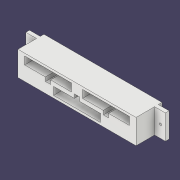
# Autodesk Inventor part: BP011
Saved by Autodesk Inventor 2017 SP1 (Build 210196100, 196)
## iProperties
Created: 2018-06-18
Part Number: BP011
Material: ABS Plastic
Document SubType Name: Modeling
Designer: Zach
Density: 1.06 g/cm^3
Appearance: CR White
Author: Zach
Autodesk Inventor part; units mm, degrees
ref_plane "YZ Plane" through (0, 0, 0) normal (1, 0, 0) x (0, 1, 0)
ref_plane "XZ Plane" through (0, 0, 0) normal (0, 1, 0) x (-1, 0, 0)
ref_plane "XY Plane" through (0, 0, 0) normal (0, 0, 1) x (1, 0, 0)
sketch "Sketch1" plane through (0, 0, 0) normal (0, 0, 1) x (1, 0, 0)
  line L0 (0, 0) -> (190, 0)
  line L1 (190, 0) -> (190, 35)
  line L2 (190, 35) -> (0, 35)
  line L3 (0, 35) -> (0, 0)
  circle A0 centre (7.5, 17.5) radius 1.5
  circle A1 centre (182.5, 17.5) radius 1.5
  point P0 (0, 17.5)
  dimension "d0" = 190
  dimension "d1" = 35
  dimension "d2" = 3
  dimension "d3" = 7.5
  dimension "d4" = 3
  dimension "d5" = 7.5
  constraints: 8 end point, 2 centre point, 2 horizontal alignment, 2 parallel, 1 horizontal, 1 midpoint, 1 perpendicular
  measures "d0" distance of L2.end L1.end
  measures "d1" distance of L1.end L0.end
  measures "d2" diameter of A0
  measures "d3" distance from line of L3 A0.centre
  measures "d4" diameter of A1
  measures "d5" distance from line of L1 A1.centre
extrude "Extrusion1" add sketch "Sketch1" along normal blind 5
sketch "Sketch2" plane through (0, 0, 0) normal (0, 0, -1) x (-1, 0, 0)
  line L0 (0, 0) -> (-190, 0) projected
  line L1 (-190, 35) -> (0, 35) projected
  line L2 (-15.5, 0) -> (-174.5, 0)
  line L3 (-174.5, 0) -> (-174.5, 35)
  line L4 (-174.5, 35) -> (-15.5, 35)
  line L5 (-15.5, 35) -> (-15.5, 0)
  point P0 (-95, 0)
  dimension "d8" = 159
  constraints: 8 end point, 2 midpoint, 2 parallel, 2 point on line, 1 horizontal, 1 perpendicular
  measures "d8" distance between parallel lines of L5 L3
extrude "Extrusion2" add sketch "Sketch2" along normal blind 5
sketch "Sketch3" plane through (0, 0, 5) normal (0, 0, 1) x (1, 0, 0)
  circle A0 centre (182.5, 17.5) radius 1.5 projected
  circle A1 centre (7.5, 17.5) radius 1.5 projected
  line L0 (0, 0) -> (190, 0) projected
  line L1 (190, 0) -> (190, 35) projected
  line L2 (190, 35) -> (0, 35) projected
  line L3 (0, 35) -> (0, 0) projected
  line L4 (1, 34) -> (189, 34)
  line L5 (189, 34) -> (189, 1)
  line L6 (189, 1) -> (1, 1)
  line L7 (1, 1) -> (1, 34)
  dimension "d11" = 1
  constraints: 8 end point, 3 other
  measures "d11" distance between parallel lines of L2 L4
extrude "Extrusion3" cut sketch "Sketch3" against normal through all contours L3 L2 L1 L0
sketch "Sketch4" plane through (0, 0, 5) normal (0, 0, 1) x (1, 0, 0)
  line L0 (41, 27) -> (71, 27)
  line L1 (71, 27) -> (71, 8)
  line L2 (71, 8) -> (41, 8)
  line L3 (41, 8) -> (41, 27)
  line L4 (86, 27) -> (116, 27)
  line L5 (116, 27) -> (116, 8)
  line L6 (116, 8) -> (86, 8)
  line L7 (86, 8) -> (86, 27)
  line L8 (131, 27) -> (149, 27)
  line L9 (149, 27) -> (149, 8)
  line L10 (149, 8) -> (131, 8)
  line L11 (131, 8) -> (131, 27)
  line L12 (41, 17.5) -> (149, 17.5) construction
  line L13 (189, 34) -> (1, 34) projected
  circle A0 centre (7.5, 17.5) radius 1.5 projected
  point P0 (0, 0)
  point P1 (95, 17.5)
  point P2 (95, 34)
  dimension "d14" = 30
  dimension "d15" = 19
  dimension "d16" = 30
  dimension "d17" = 19
  dimension "d18" = 18
  dimension "d19" = 19
  dimension "d20" = 15
  dimension "d21" = 15
  constraints: 26 end point, 6 parallel, 4 midpoint, 3 horizontal, 3 perpendicular, 2 point on line, 1 horizontal alignment, 1 vertical alignment
  measures "d14" distance of L1.end L2.end
  measures "d15" distance of L0.end L1.end
  measures "d16" distance of L5.end L6.end
  measures "d17" distance of L4.end L5.end
  measures "d18" distance of L9.end L10.end
  measures "d19" distance of L8.end L9.end
  measures "d20" distance between parallel lines of L1 L7
  measures "d21" distance between parallel lines of L11 L5
extrude "Extrusion4" cut sketch "Sketch4" against normal through all contours L0 L1 L2 L3 | L4 L5 L6 L7 | L8 L9 L10 L11
sketch "Sketch5" plane through (0, 0, 5) normal (0, 0, 1) x (1, 0, 0)
  line L0 (41, 27) -> (41, 8) projected
  line L1 (41, 8) -> (71, 8) projected
  line L2 (71, 8) -> (71, 27) projected
  line L3 (71, 27) -> (41, 27) projected
  line L4 (131, 27) -> (131, 8) projected
  line L5 (131, 8) -> (149, 8) projected
  line L6 (149, 8) -> (149, 27) projected
  line L7 (149, 27) -> (131, 27) projected
  line L8 (86, 27) -> (86, 8) projected
  line L9 (86, 8) -> (116, 8) projected
  line L10 (116, 8) -> (116, 27) projected
  line L11 (116, 27) -> (86, 27) projected
  line L12 (174.5, 1) -> (15.5, 1) projected
  line L13 (15.5, 1) -> (15.5, 34) projected
  line L14 (15.5, 34) -> (174.5, 34) projected
  line L15 (174.5, 34) -> (174.5, 1) projected
  point P0 (0, 0)
extrude "Extrusion5" add sketch "Sketch5" along normal blind 25
sketch "Sketch6" plane through (0, 0, -5) normal (0, 0, -1) x (-1, 0, 0)
  line L0 (-71, 27) -> (-41, 27) projected
  line L1 (-41, 27) -> (-41, 8) projected
  line L2 (-71, 8) -> (-71, 27) projected
  line L3 (-86, 27) -> (-86, 8) projected
  line L4 (-116, 27) -> (-86, 27) projected
  line L5 (-116, 8) -> (-116, 27) projected
  line L6 (-41, 25) -> (-36, 25)
  line L7 (-36, 25) -> (-36, 10)
  line L8 (-36, 10) -> (-41, 10)
  line L9 (-41, 10) -> (-41, 25)
  line L10 (-71, 25) -> (-76, 25)
  line L11 (-76, 25) -> (-76, 10)
  line L12 (-76, 10) -> (-71, 10)
  line L13 (-71, 10) -> (-71, 25)
  line L14 (-86, 25) -> (-81, 25)
  line L15 (-81, 25) -> (-81, 10)
  line L16 (-81, 10) -> (-86, 10)
  line L17 (-86, 10) -> (-86, 25)
  line L18 (-116, 25) -> (-121, 25)
  line L19 (-121, 25) -> (-121, 10)
  line L20 (-121, 10) -> (-116, 10)
  line L21 (-116, 10) -> (-116, 25)
  point P0 (0, 0)
  point P1 (-41, 17.5)
  dimension "d26" = 15
  dimension "d27" = 5
  dimension "d28" = 5
  dimension "d29" = 5
  dimension "d30" = 5
  constraints: 32 end point, 8 parallel, 6 horizontal alignment, 4 horizontal, 4 perpendicular, 4 point on line, 2 midpoint
  measures "d26" distance of L6.end L7.end
  measures "d27" distance of L6.start L6.end
  measures "d28" distance of L10.start L10.end
  measures "d29" distance of L14.start L14.end
  measures "d30" distance of L18.start L18.end
extrude "Extrusion6" cut sketch "Sketch6" against normal blind 22
sketch "Sketch10" plane through (0, 0, 30) normal (0, 0, 1) x (1, 0, 0)
  line L0 (86, 27) -> (116, 27) projected
  line L1 (116, 27) -> (116, 8) projected
  line L2 (116, 8) -> (86, 8) projected
  line L3 (86, 8) -> (86, 27) projected
  line L4 (41, 27) -> (71, 27) projected
  line L5 (71, 27) -> (71, 8) projected
  line L6 (71, 8) -> (41, 8) projected
  line L7 (41, 8) -> (41, 27) projected
  line L8 (131, 27) -> (149, 27) projected
  line L9 (149, 27) -> (149, 8) projected
  line L10 (149, 8) -> (131, 8) projected
  line L11 (131, 8) -> (131, 27) projected
  line L12 (15.5, 1) -> (174.5, 1) projected
  line L13 (174.5, 1) -> (174.5, 34) projected
  line L14 (174.5, 34) -> (15.5, 34) projected
  line L15 (15.5, 34) -> (15.5, 1) projected
  point P0 (0, 0)
extrude "Extrusion7" add sketch "Sketch10" against normal blind 35 contours L0 L1 L2 L3 | L4 L5 L6 L7 | L8 L9 L10 L11 | L15 L14 L13 L12
sketch "Sketch11" plane through (0, 0, 30) normal (0, 0, 1) x (1, 0, 0)
  line L0 (29.5, 32) -> (82.5, 32)
  line L1 (82.5, 32) -> (82.5, 19)
  line L2 (82.5, 19) -> (29.5, 19)
  line L3 (29.5, 19) -> (29.5, 32)
  line L4 (107.5, 32) -> (160.5, 32)
  line L5 (160.5, 32) -> (160.5, 19)
  line L6 (160.5, 19) -> (107.5, 19)
  line L7 (107.5, 19) -> (107.5, 32)
  line L8 (29.5, 32) -> (160.5, 32)
  line L9 (174.5, 34) -> (15.5, 34) projected
  line L10 (29.5, 32) -> (29.5, 3)
  line L11 (15.5, 34) -> (15.5, 1) projected
  line L12 (52.5, 19) -> (59.5, 19)
  line L13 (59.5, 19) -> (59.5, 15)
  line L14 (59.5, 15) -> (52.5, 15)
  line L15 (52.5, 15) -> (52.5, 19)
  line L16 (130.5, 19) -> (137.5, 19)
  line L17 (137.5, 19) -> (137.5, 15)
  line L18 (137.5, 15) -> (130.5, 15)
  line L19 (130.5, 15) -> (130.5, 19)
  line L20 (68.5, 3) -> (121.5, 3)
  line L21 (121.5, 3) -> (121.5, 16)
  line L22 (121.5, 16) -> (68.5, 16)
  line L23 (68.5, 16) -> (68.5, 3)
  line L24 (91.5, 16) -> (98.5, 16)
  line L25 (98.5, 16) -> (98.5, 20)
  line L26 (98.5, 20) -> (91.5, 20)
  line L27 (91.5, 20) -> (91.5, 16)
  point P0 (0, 0)
  point P1 (95, 32)
  point P2 (95, 34)
  point P3 (29.5, 17.5)
  point P4 (15.5, 17.5)
  point P5 (56, 19)
  point P6 (134, 19)
  point P7 (95, 16)
  point P8 (95, 20)
  dimension "d40" = 53
  dimension "d41" = 13
  dimension "d42" = 53
  dimension "d43" = 13
  dimension "d46" = 25
  dimension "d48" = 7
  dimension "d49" = 7
  dimension "d50" = 4
  dimension "d53" = 53
  dimension "d54" = 13
  dimension "d55" = 7
  dimension "d56" = 4
  dimension "d57" = 3
  dimension "d58" = 4
  constraints: 52 end point, 12 parallel, 11 midpoint, 6 horizontal, 6 perpendicular, 4 point on line, 3 horizontal alignment, 2 vertical alignment
  measures "d40" distance of L1.end L2.end
  measures "d41" distance of L2.end L0.start
  measures "d42" distance of L5.end L6.end
  measures "d43" distance of L6.end L4.start
  measures "d46" distance between parallel lines of L7 L1
  measures "d48" distance between parallel lines of L15 L13
  measures "d49" distance of L17.end L18.end
  measures "d50" distance of L16.end L17.end
  measures "d53" distance of L22.end L21.end
  measures "d54" distance of L21.end L20.end
  measures "d55" distance of L26.end L25.end
  measures "d56" distance of L25.end L24.end
  measures "d57" distance between parallel lines of L2 L22
  measures "d58" distance of L14.end L12.start
extrude "Extrusion8" cut sketch "Sketch11" against normal through all
sketch "Sketch13" plane through (0, 0, 30) normal (0, 0, 1) x (1, 0, 0)
  line L0 (98.5, 16) -> (121.5, 16) projected
  line L1 (121.5, 16) -> (121.5, 3) projected
  line L2 (121.5, 3) -> (68.5, 3) projected
  line L3 (68.5, 3) -> (68.5, 16) projected
  line L4 (68.5, 16) -> (91.5, 16) projected
  line L5 (91.5, 16) -> (91.5, 20) projected
  line L6 (91.5, 20) -> (98.5, 20) projected
  line L7 (98.5, 20) -> (98.5, 16) projected
  line L8 (52.5, 19) -> (29.5, 19) projected
  line L9 (29.5, 19) -> (29.5, 32) projected
  line L10 (29.5, 32) -> (82.5, 32) projected
  line L11 (82.5, 32) -> (82.5, 19) projected
  line L12 (82.5, 19) -> (59.5, 19) projected
  line L13 (59.5, 19) -> (59.5, 15) projected
  line L14 (59.5, 15) -> (52.5, 15) projected
  line L15 (52.5, 15) -> (52.5, 19) projected
  line L16 (130.5, 19) -> (107.5, 19) projected
  line L17 (107.5, 19) -> (107.5, 32) projected
  line L18 (107.5, 32) -> (160.5, 32) projected
  line L19 (160.5, 32) -> (160.5, 19) projected
  line L20 (160.5, 19) -> (137.5, 19) projected
  line L21 (137.5, 19) -> (137.5, 15) projected
  line L22 (137.5, 15) -> (130.5, 15) projected
  line L23 (130.5, 15) -> (130.5, 19) projected
  line L24 (15.5, 1) -> (174.5, 1) projected
  line L25 (174.5, 1) -> (174.5, 34) projected
  line L26 (174.5, 34) -> (15.5, 34) projected
  line L27 (15.5, 34) -> (15.5, 1) projected
  point P0 (0, 0)
extrude "Extrusion10" cut sketch "Sketch13" against normal blind 25
sketch "Sketch12" plane through (0, 0, 5) normal (0, 0, 1) x (1, 0, 0)
  line L0 (29.5, 19) -> (29.5, 32)
  line L1 (82.5, 32) -> (82.5, 19)
  line L2 (29.5, 30.75) -> (82.5, 30.75)
  line L3 (82.5, 30.75) -> (82.5, 20.25)
  line L4 (82.5, 20.25) -> (29.5, 20.25)
  line L5 (29.5, 20.25) -> (29.5, 30.75)
  line L6 (107.5, 19) -> (107.5, 32)
  line L7 (160.5, 19) -> (160.5, 32)
  line L8 (107.5, 30.75) -> (160.5, 30.75)
  line L9 (160.5, 30.75) -> (160.5, 20.25)
  line L10 (160.5, 20.25) -> (107.5, 20.25)
  line L11 (107.5, 20.25) -> (107.5, 30.75)
  line L12 (121.5, 3) -> (121.5, 16)
  line L13 (121.5, 14.75) -> (68.5, 14.75)
  line L14 (68.5, 14.75) -> (68.5, 4.25)
  line L15 (68.5, 4.25) -> (121.5, 4.25)
  line L16 (121.5, 4.25) -> (121.5, 14.75)
  line L17 (68.5, 3) -> (68.5, 16)
  line L18 (98.5, 16) -> (121.5, 16)
  line L19 (121.5, 16) -> (121.5, 3)
  line L20 (121.5, 3) -> (68.5, 3)
  line L21 (68.5, 3) -> (68.5, 16)
  line L22 (68.5, 16) -> (91.5, 16)
  line L23 (91.5, 16) -> (91.5, 20)
  line L24 (91.5, 20) -> (98.5, 20)
  line L25 (98.5, 20) -> (98.5, 16)
  line L26 (52.5, 19) -> (29.5, 19)
  line L27 (29.5, 19) -> (29.5, 32)
  line L28 (29.5, 32) -> (82.5, 32)
  line L29 (82.5, 32) -> (82.5, 19)
  line L30 (82.5, 19) -> (59.5, 19)
  line L31 (59.5, 19) -> (59.5, 15)
  line L32 (59.5, 15) -> (52.5, 15)
  line L33 (52.5, 15) -> (52.5, 19)
  line L34 (130.5, 19) -> (107.5, 19)
  line L35 (107.5, 19) -> (107.5, 32)
  line L36 (107.5, 32) -> (160.5, 32)
  line L37 (160.5, 32) -> (160.5, 19)
  line L38 (160.5, 19) -> (137.5, 19)
  line L39 (137.5, 19) -> (137.5, 15)
  line L40 (137.5, 15) -> (130.5, 15)
  line L41 (130.5, 15) -> (130.5, 19)
  line L42 (15.5, 1) -> (174.5, 1)
  line L43 (174.5, 1) -> (174.5, 34)
  line L44 (174.5, 34) -> (15.5, 34)
  line L45 (15.5, 34) -> (15.5, 1)
  line L46 (98.5, 16) -> (98.5, 20)
  line L47 (91.5, 14.75) -> (98.5, 14.75)
  line L48 (98.5, 14.75) -> (98.5, 20)
  line L49 (98.5, 20) -> (91.5, 20)
  line L50 (91.5, 20) -> (91.5, 14.75)
  line L51 (52.5, 19) -> (52.5, 15)
  line L52 (52.5, 15) -> (59.5, 15)
  line L53 (59.5, 15) -> (59.5, 20.25)
  line L54 (59.5, 20.25) -> (52.5, 20.25)
  line L55 (52.5, 20.25) -> (52.5, 15)
  line L56 (130.5, 15) -> (137.5, 15)
  line L57 (130.5, 15) -> (137.5, 15)
  line L58 (137.5, 15) -> (137.5, 20.25)
  line L59 (137.5, 20.25) -> (130.5, 20.25)
  line L60 (130.5, 20.25) -> (130.5, 15)
  point P0 (0, 0)
  point P1 (68.5, 9.5)
  point P2 (121.5, 9.5)
  point P3 (29.5, 25.5)
  point P4 (160.5, 25.5)
  point P5 (107.5, 25.5)
  dimension "d59" = 10.5
  dimension "d60" = 10.5
  constraints: 122 end point, 13 point on line, 12 parallel, 10 midpoint, 6 horizontal, 6 perpendicular
  measures "d59" distance between parallel lines of L4 L2
  measures "d60" distance between parallel lines of L15 L13
extrude "Extrusion9" add sketch "Sketch12" against normal blind 3 contours L0 L4 L55 L26 | L0 L28 L1 L2 | L4 L1 L30 L53 | L6 L10 L60 L34 | L6 L36 L7 L8 | L10 L7 L38 L58 | L20 L17 L15 L12 | L13 L48 L18 L12 | L17 L22 L50 L13
sketch "Sketch14" plane through (0, 0, 5) normal (0, 0, 1) x (1, 0, 0)
  line L0 (15.5, 34) -> (15.5, 1) projected
  line L1 (174.5, 1) -> (174.5, 34) projected
  circle A0 centre (7.5, 17.5) radius 1.5 projected
  line L2 (130.5, 20.25) -> (130.5, 15) projected
  line L3 (130.5, 20.25) -> (107.5, 20.25) projected
  line L4 (107.5, 30.75) -> (107.5, 20.25) projected
  line L5 (107.5, 30.75) -> (160.5, 30.75) projected
  line L6 (160.5, 20.25) -> (160.5, 30.75) projected
  line L7 (160.5, 20.25) -> (137.5, 20.25) projected
  line L8 (137.5, 20.25) -> (137.5, 15) projected
  line L9 (130.5, 15) -> (137.5, 15) projected
  line L10 (52.5, 20.25) -> (52.5, 15) projected
  line L11 (52.5, 20.25) -> (29.5, 20.25) projected
  line L12 (29.5, 30.75) -> (29.5, 20.25) projected
  line L13 (29.5, 30.75) -> (82.5, 30.75) projected
  line L14 (82.5, 20.25) -> (82.5, 30.75) projected
  line L15 (82.5, 20.25) -> (59.5, 20.25) projected
  line L16 (59.5, 20.25) -> (59.5, 15) projected
  line L17 (52.5, 15) -> (59.5, 15) projected
  line L18 (98.5, 14.75) -> (98.5, 20) projected
  line L19 (98.5, 14.75) -> (121.5, 14.75) projected
  line L20 (121.5, 4.25) -> (121.5, 14.75) projected
  line L21 (121.5, 4.25) -> (68.5, 4.25) projected
  line L22 (68.5, 14.75) -> (68.5, 4.25) projected
  line L23 (68.5, 14.75) -> (91.5, 14.75) projected
  line L24 (91.5, 14.75) -> (91.5, 20) projected
  line L25 (98.5, 20) -> (91.5, 20) projected
  circle A1 centre (182.5, 17.5) radius 1.5 projected
  line L26 (1, 1) -> (189, 1) projected
  line L27 (189, 1) -> (189, 34) projected
  line L28 (189, 34) -> (1, 34) projected
  line L29 (1, 34) -> (1, 1) projected
  line L30 (29.5, 30.75) -> (29.5, 20.25) projected
  line L31 (29.5, 30.75) -> (24.5, 30.75)
  line L32 (24.5, 30.75) -> (24.5, 20.25)
  line L33 (24.5, 20.25) -> (29.5, 20.25)
  line L34 (29.5, 20.25) -> (29.5, 30.75)
  line L35 (121.5, 14.75) -> (126.5, 14.75)
  line L36 (126.5, 14.75) -> (126.5, 4.25)
  line L37 (126.5, 4.25) -> (121.5, 4.25)
  line L38 (121.5, 4.25) -> (121.5, 14.75)
  line L39 (160.5, 20.25) -> (160.5, 30.75) projected
  line L40 (160.5, 30.75) -> (165.5, 30.75)
  line L41 (165.5, 30.75) -> (165.5, 20.25)
  line L42 (165.5, 20.25) -> (160.5, 20.25)
  line L43 (160.5, 20.25) -> (160.5, 30.75)
  line L44 (107.5, 30.75) -> (107.5, 20.25) projected
  line L45 (107.5, 30.75) -> (102.5, 30.75)
  line L46 (102.5, 30.75) -> (102.5, 20.25)
  line L47 (102.5, 20.25) -> (107.5, 20.25)
  line L48 (107.5, 20.25) -> (107.5, 30.75)
  line L49 (82.5, 30.75) -> (87.5, 30.75)
  line L50 (87.5, 30.75) -> (87.5, 20.25)
  line L51 (87.5, 20.25) -> (82.5, 20.25)
  line L52 (82.5, 20.25) -> (82.5, 30.75)
  line L53 (68.5, 14.75) -> (63.5, 14.75)
  line L54 (63.5, 14.75) -> (63.5, 4.25)
  line L55 (63.5, 4.25) -> (68.5, 4.25)
  line L56 (68.5, 4.25) -> (68.5, 14.75)
  line L57 (1, 34) -> (15.5, 34) projected
  line L58 (1, 34) -> (15.5, 34)
  line L59 (15.5, 34) -> (15.5, 1)
  line L60 (15.5, 1) -> (1, 1)
  line L61 (1, 1) -> (1, 34)
  line L62 (174.5, 1) -> (189, 1)
  line L63 (189, 1) -> (189, 34)
  line L64 (189, 34) -> (174.5, 34)
  line L65 (174.5, 34) -> (174.5, 1)
  point P0 (0, 0)
  dimension "d65" = 5
  dimension "d66" = 5
  dimension "d67" = 5
  dimension "d68" = 5
  dimension "d69" = 5
  dimension "d70" = 5
  constraints: 64 end point, 16 parallel, 8 horizontal, 8 perpendicular, 2 point on line
  measures "d65" distance of L11.end L32.end
  measures "d66" distance of L20.start L36.end
  measures "d67" distance of L6.start L41.end
  measures "d68" distance of L47.end L46.end
  measures "d69" distance of L14.start L50.end
  measures "d70" distance of L55.end L54.end
extrude "Extrusion12" add sketch "Sketch14" along normal blind 25 contours L28 L1 L26 L0
body "Solid1"
